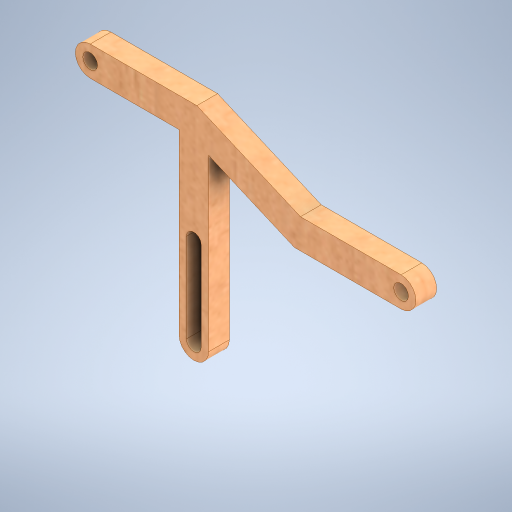
# Autodesk Inventor part: BrazoV2
Saved by Autodesk Inventor 2023.1 (Build 271208000, 208)
## iProperties
Created: 2022-10-30
Part Number: BrazoV2
Material: MDF Medium Density Fiberboard
Document SubType Name: Modeling
Designer: Daniel Peña
Density: 0.8 g/cm^3
Appearance: Cherry - Natural Low Gloss
Author: Daniel Peña
Autodesk Inventor part; units mm, degrees
ref_plane "YZ Plane" through (0, 0, 0) normal (1, 0, 0) x (0, 1, 0)
ref_plane "XZ Plane" through (0, 0, 0) normal (0, 1, 0) x (-1, 0, 0)
ref_plane "XY Plane" through (0, 0, 0) normal (0, 0, 1) x (1, 0, 0)
sketch "Sketch1" plane through (0, 0, 0) normal (0, 0, 1) x (1, 0, 0)
  line L0 (-16.7246, 10.0225) -> (18.2754, 10.0225) construction
  line L1 (53.2754, -4.9775) -> (88.2754, -4.9775) construction
  line L2 (18.2754, 10.0225) -> (53.2754, -4.9775) construction
  line L3 (-16.7246, 15.0225) -> (19.3017, 15.0225)
  line L4 (19.3017, 15.0225) -> (54.3017, 0.0225)
  line L5 (54.3017, 0.0225) -> (88.2754, 0.0225)
  line L6 (-16.7246, 5.0225) -> (13.2754, 5.0225)
  line L7 (52.2491, -9.9775) -> (88.2754, -9.9775)
  line L8 (-21.7246, 10.0225) -> (-21.7246, 10.0225)
  line L9 (93.2754, -4.9775) -> (93.2754, -4.9775)
  line L10 (18.2754, 10.0225) -> (18.2754, -54.9775) construction
  line L11 (23.2754, 2.4398) -> (23.2754, -54.9775)
  line L12 (18.2754, -59.9775) -> (18.2754, -59.9775)
  line L13 (13.2754, -54.9775) -> (13.2754, 5.0225)
  line L14 (23.2754, 2.4398) -> (52.2491, -9.9775)
  arc A0 (-21.7246, 10.0225) -> (-16.7246, 5.0225) centre (-16.7246, 10.0225) ccw
  arc A1 (-16.7246, 15.0225) -> (-21.7246, 10.0225) centre (-16.7246, 10.0225) ccw
  arc A2 (93.2754, -4.9775) -> (88.2754, 0.0225) centre (88.2754, -4.9775) ccw
  arc A3 (88.2754, -9.9775) -> (93.2754, -4.9775) centre (88.2754, -4.9775) ccw
  arc A4 (18.2754, -59.9775) -> (23.2754, -54.9775) centre (18.2754, -54.9775) ccw
  arc A5 (13.2754, -54.9775) -> (18.2754, -59.9775) centre (18.2754, -54.9775) ccw
  point P0 (0, 0)
  dimension "d0" = 35
  dimension "d4" = 35
  dimension "d5" = 35
  dimension "d6" = 15
  dimension "d7" = 5
  dimension "d8" = 5
  dimension "d10" = 5
  dimension "d11" = 5
  dimension "d13" = 65
  dimension "d14" = 5
  dimension "d15" = 5
  dimension "d16" = 5
  constraints: 30 end point, 12 point on circle, 12 tangent, 6 centre point, 5 equal radius, 3 vertical, 1 horizontal, 1 parallel, 1 other
  measures "d0" distance of L0.start L0.end
  measures "d4" distance of L1.start L1.end
  measures "d5" horizontal distance of L1.start L0.end
  measures "d6" vertical distance of L1.start L0.end
  measures "d7" distance between parallel lines of L0 L3
  measures "d8" distance between parallel lines of L0 L6
  measures "d10" distance from line of L0.start L8
  measures "d11" distance from line of L9 L1.end
  measures "d13" distance of L0.end L10.end
  measures "d14" distance between parallel lines of L11 L10
  measures "d15" distance from line of L10.end L12
  measures "d16" radius of A0
extrude "Extrusion1" add sketch "Sketch1" along normal blind 7
sketch "Sketch2" plane through (0, 0, 7) normal (0, 0, 1) x (1, 0, 0)
  arc A0 (-16.7246, 15.0225) -> (-16.7246, 5.0225) centre (-16.7246, 10.0225) ccw projected
  arc A1 (88.2754, -9.9775) -> (88.2754, 0.0225) centre (88.2754, -4.9775) ccw projected
  point P0 (0, 0)
  constraints: 2 coincident
hole "Hole1" at (-16.7246, 10.0225, 7) at (88.2754, -4.9775, 7) direction (0, 0, -1) diameter 5 end through all
sketch "Sketch3" plane through (0, 0, 7) normal (0, 0, 1) x (1, 0, 0)
  arc A0 (13.2754, -54.9775) -> (23.2754, -54.9775) centre (18.2754, -54.9775) ccw construction
  line L0 (18.2754, -54.9775) -> (18.2754, -24.9775) construction
  line L1 (18.2754, -22.4775) -> (18.2754, -22.4775)
  line L2 (20.7754, -24.9775) -> (20.7754, -54.9775)
  line L3 (18.2754, -57.4775) -> (18.2754, -57.4775)
  line L4 (15.7754, -54.9775) -> (15.7754, -24.9775)
  arc A1 (18.2754, -22.4775) -> (15.7754, -24.9775) centre (18.2754, -24.9775) ccw
  arc A2 (20.7754, -24.9775) -> (18.2754, -22.4775) centre (18.2754, -24.9775) ccw
  arc A3 (15.7754, -54.9775) -> (18.2754, -57.4775) centre (18.2754, -54.9775) ccw
  arc A4 (18.2754, -57.4775) -> (20.7754, -54.9775) centre (18.2754, -54.9775) ccw
  point P0 (0, 0)
  dimension "d26" = 30
  dimension "d28" = 2.5
  dimension "d29" = 2.5
  dimension "d30" = 2.5
  dimension "d31" = 2.5
  constraints: 10 end point, 8 point on circle, 8 tangent, 4 centre point, 3 equal radius, 2 parallel, 1 horizontal, 1 perpendicular, 1 vertical, 1 other
  measures "d26" distance of L0.start L0.end
  measures "d28" distance from line of L1 L0.end
  measures "d29" distance from line of L0.start L3
  measures "d30" distance between parallel lines of L4 L0
  measures "d31" radius of A1
extrude "Extrusion2" cut sketch "Sketch3" against normal blind 7
body "Solid1"
